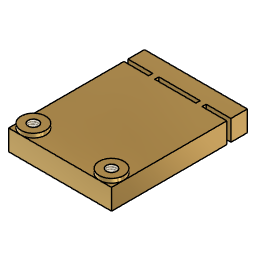
frog polisher final draft (Autodesk Fusion 360 design; units mm, degrees)
Autodesk Fusion 360 part; units mm, degrees
sketch "Sketch1" plane through (0, 0, 0) normal (0, 0, 1) x (1, 0, 0)
  line L0 (0, 0) -> (50, 0)
  line L1 (50, 0) -> (50, 56)
  line L2 (50, 56) -> (0, 56)
  line L3 (0, 56) -> (0, 0)
  dimension "d1" = 50
  dimension "d2" = 56
  constraint horizontal L0
  constraint vertical L1
  constraint horizontal L2
  constraint vertical L3
  constraint coincident L0.start L3.end
  measures "d1" distance of L0.start L0.end
  measures "d2" distance of L0.start L2.end
extrude "Extrude1" add sketch "Sketch1" along normal blind 10
sketch "Sketch2" plane through (0, 0, 10) normal (0, 0, 1) x (-1, 0, 0)
  line L0 (0, -56) -> (0, 0)
  line L1 (0, 0) -> (-50, 0)
  line L2 (-50, 0) -> (-50, -56)
  line L3 (-50, -56) -> (0, -56)
  line L4 (0, 0) -> (-6, 0)
  line L5 (-6, 0) -> (-6, -6)
  circle A0 centre (-6, -6) radius 6
  line L6 (-50, 0) -> (-44, 0)
  line L7 (-44, 0) -> (-44, -6)
  circle A1 centre (-44, -6) radius 6
  dimension "d5" = 6
  dimension "d6" = 6
  dimension "d7" = 12
  dimension "d8" = 6
  dimension "d9" = 6
  dimension "d10" = 12
  constraint coincident L0.end L1.start
  constraint coincident L1 L4.end
  constraint perpendicular L4 L5
  constraint coincident L5.end A0.centre
  constraint coincident L1.end L2.start
  constraint perpendicular L2 L6
  constraint perpendicular L6 L7
  constraint coincident L7.end A1.centre
  measures "d5" distance of L0.end L4.end
  measures "d6" distance of L4.end L5.end
  measures "d7" diameter of A0
  measures "d8" distance of L1.end L6.end
  measures "d9" distance of L6.end L7.end
  measures "d10" diameter of A1
extrude "Extrude2" add sketch "Sketch2" along normal blind 2 contours A0 | A1
sketch "Sketch3" plane through (0, 0, 12) normal (0, 0, 1) x (-1, 0, 0)
  circle A0 centre (-6, -6) radius 6
  line L0 (-6, -6) -> (-12, -6)
  constraint coincident A0.centre L0.start
  constraint coincident A0 L0.end
  constraint horizontal L0
sketch "Sketch4" plane through (0, 0, 12) normal (0, 0, 1) x (-1, 0, 0)
  circle A0 centre (-44, -6) radius 6
  line L0 (-44, -6) -> (-50, -6)
  constraint coincident A0.centre L0.start
  constraint coincident A0 L0.end
  constraint horizontal L0
hole "Hole1" at (6, 6, 12) at (44, 6, 12) direction (0, 0, -1) diameter 5.035 depth 15 tip angle 118
thread "Thread1" "ISO Metric profile 6.0 M6x1 6H"
sketch "Sketch5" plane through (0, 56, 0) normal (0, 1, 0) x (-1, 0, 0)
  line L0 (-50, 0) -> (0, 0)
  line L1 (0, 0) -> (0, 10)
  line L2 (0, 10) -> (-50, 10)
  line L3 (-50, 10) -> (-50, 0)
  line L4 (-50, 5) -> (-45, 5)
  line L5 (0, 5) -> (-5, 5)
  dimension "d23" = 5
  dimension "d24" = 5
  constraint midpoint L3 L4.start
  constraint perpendicular L3 L4
  constraint midpoint L1 L5.start
  constraint perpendicular L1 L5
  measures "d23" distance of L4.start L4.end
  measures "d24" distance of L5.start L5.end
hole "Hole3" at (45, 56, 5) at (5, 56, 5) direction (0, -1, 0) diameter 5.035 depth 18 tip angle 118
thread "Thread3" "ISO Metric profile 6.0 M6x1 6H"
sketch "Sketch6" plane through (0, 56, 0) normal (0, 1, 0) x (-1, 0, 0)
  circle A0 centre (-45, 5) radius 2.5175
  circle A1 centre (-5, 5) radius 2.5175
  line L0 (-50, 0) -> (0, 0)
  line L1 (0, 0) -> (0, 10)
  line L2 (0, 10) -> (-50, 10)
  line L3 (-50, 10) -> (-50, 0)
  line L4 (-45, 5) -> (-35, 5)
  line L5 (-5, 5) -> (-15, 5)
  line L6 (-35, 5) -> (-35, 0)
  line L7 (-15, 5) -> (-15, 0)
  line L8 (-35, 0) -> (-38, 0)
  line L9 (-38, 0) -> (-38, 10)
  line L10 (-38, 10) -> (-35, 10)
  line L11 (-35, 10) -> (-35, 0)
  line L12 (-15, 0) -> (-12, 0)
  line L13 (-12, 0) -> (-12, 10)
  line L14 (-12, 10) -> (-15, 10)
  line L15 (-15, 10) -> (-15, 0)
  dimension "d28" = 10
  dimension "d29" = 10
  dimension "d30" = 3
  dimension "d31" = 3
  constraint coincident A0.centre L4.start
  constraint horizontal L4
  constraint coincident A1.centre L5.start
  constraint parallel L2 L5
  constraint coincident L0 L6.end
  constraint perpendicular L0 L6
  constraint coincident L0 L7.end
  constraint perpendicular L0 L7
  constraint horizontal L8
  constraint vertical L9
  constraint horizontal L10
  constraint vertical L11
  constraint coincident L2 L9.end
  constraint horizontal L12
  constraint vertical L13
  constraint horizontal L14
  constraint vertical L15
  constraint coincident L2 L13.end
  measures "d28" distance of A0.centre L4.end
  measures "d29" distance of A1.centre L5.end
  measures "d30" distance of L6.end L8.end
  measures "d31" distance of L7.end L12.end
extrude "Extrude3" add sketch "Sketch6" along normal blind 2 contours L0 L4 L6 L8 L9 L11 | L2 L4 L9 L10 L11 | L0 L5 L7 L12 L13 L15 | L2 L5 L13 L14 L15
sketch "Sketch7" plane through (0, 58, 0) normal (0, 1, 0) x (-1, 0, 0)
  line L0 (-35, 10) -> (-38, 10)
  line L1 (-38, 10) -> (-38, 0)
  line L2 (-38, 0) -> (-35, 0)
  line L3 (-35, 0) -> (-35, 10)
  line L4 (-35, 0) -> (-50, 0)
  line L5 (-50, 0) -> (-50, 10)
  line L6 (-50, 10) -> (-35, 10)
  line L7 (-35, 10) -> (-35, 0)
  line L8 (-35, 0) -> (0, 0)
  line L9 (0, 0) -> (0, 10)
  line L10 (0, 10) -> (-35, 10)
  line L11 (-35, 10) -> (-35, 0)
  dimension "d34" = 15
  dimension "d35" = 10
  dimension "d36" = 35
  dimension "d37" = 10
  constraint horizontal L4
  constraint vertical L5
  constraint horizontal L6
  constraint vertical L7
  constraint coincident L2.end L3.start
  constraint horizontal L8
  constraint vertical L9
  constraint horizontal L10
  constraint vertical L11
  measures "d34" distance of L2.end L4.end
  measures "d35" distance of L2.end L0.start
  measures "d36" distance of L2.end L8.end
  measures "d37" distance of L2.end L0.start
extrude "Extrude4" add sketch "Sketch7" along normal blind 8
sketch "Sketch8" plane through (0, 66, 0) normal (0, 1, 0) x (-1, 0, 0)
  line L0 (-50, 0) -> (0, 0)
  line L1 (0, 0) -> (0, 10)
  line L2 (0, 10) -> (-50, 10)
  line L3 (-50, 10) -> (-50, 0)
  line L4 (-50, 5) -> (-45, 5)
  line L5 (0, 5) -> (-5, 5)
  dimension "d40" = 5
  dimension "d41" = 5
  constraint midpoint L3 L4.start
  constraint perpendicular L3 L4
  constraint midpoint L1 L5.start
  constraint perpendicular L1 L5
  measures "d40" distance of L4.start L4.end
  measures "d41" distance of L5.start L5.end
hole "Hole4" at (45, 66, 5) at (5, 66, 5) direction (0, -1, 0) diameter 5.035 depth 28 tip angle 118
thread "Thread4" "ISO Metric profile 6.0 M6x1 6H"
